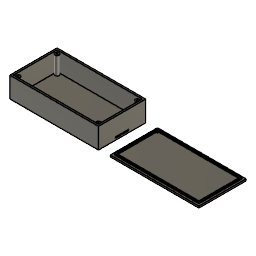
caja sensor examen (Autodesk Fusion 360 design; units mm, degrees)
part number: 2026-07-09-18-08-44-658
Autodesk Fusion 360 part; units mm, degrees
note: some values were not read from the file. Chosen so that the rebuilt part matches the saved one: which bodies a step acts on.
sketch "Boceto1" plane through (0, 0, 0) normal (0, 0, 1) x (1, 0, 0)
  line L0 (0, 0) -> (150, 0)
  line L1 (150, 0) -> (150, 80)
  line L2 (150, 80) -> (0, 80)
  line L3 (0, 80) -> (0, 0)
extrude "Extruir1" add sketch "Boceto1" along normal blind 3 makes body 1
sketch "Boceto2" plane through (0, 0, 0) normal (0, 0, 1) x (1, 0, 0)
  line L0 (0, 0) -> (150, 0)
  line L1 (150, 0) -> (150, 3)
  line L2 (150, 3) -> (0, 3)
  line L3 (0, 3) -> (0, 0)
extrude "Extruir2" add sketch "Boceto2" along normal blind 32 separate body makes body 2
move_body "Desplazar1" bodies 2 to x (1, 0, 0) y (0, 1, 0) z (0, 0, 1) at (0, 0, 3)
sketch "Boceto3" plane through (0, 0, 0) normal (0, 0, 1) x (1, 0, 0)
  line L0 (0, 77) -> (150, 77)
  line L1 (150, 77) -> (150, 80)
  line L2 (150, 80) -> (0, 80)
  line L3 (0, 80) -> (0, 77)
extrude "Extruir3" add sketch "Boceto3" along normal blind 32 separate body makes body 3
move_body "Desplazar2" bodies 3 to x (1, 0, 0) y (0, 1, 0) z (0, 0, 1) at (0, 0, 3)
sketch "Boceto4" plane through (0, 0, 0) normal (0, 0, 1) x (1, 0, 0)
  line L0 (0, 0) -> (3, 0)
  line L1 (3, 0) -> (3, 80)
  line L2 (3, 80) -> (0, 80)
  line L3 (0, 80) -> (0, 0)
extrude "Extruir4" add sketch "Boceto4" along normal blind 32 separate body makes body 4
move_body "Desplazar3" bodies 4 to x (1, 0, 0) y (0, 1, 0) z (0, 0, 1) at (0, 0, 3)
sketch "Boceto5" plane through (0, 0, 0) normal (0, 0, 1) x (1, 0, 0)
  line L0 (147, 0) -> (150, 0)
  line L1 (150, 0) -> (150, 29)
  line L2 (150, 29) -> (147, 29)
  line L3 (147, 29) -> (147, 0)
extrude "Extruir5" add sketch "Boceto5" along normal blind 32 separate body makes body 5
move_body "Desplazar4" bodies 5 to x (1, 0, 0) y (0, 1, 0) z (0, 0, 1) at (0, 0, 3)
sketch "Boceto6" plane through (0, 0, 0) normal (0, 0, 1) x (1, 0, 0)
  line L0 (147, 39) -> (150, 39)
  line L1 (150, 39) -> (150, 41)
  line L2 (150, 41) -> (147, 41)
  line L3 (147, 41) -> (147, 39)
extrude "Extruir6" add sketch "Boceto6" along normal blind 2 separate body makes body 6
move_body "Desplazar5" bodies 6 to x (1, 0, 0) y (0, 1, 0) z (0, 0, 1) at (0, 0, 3)
sketch "Boceto7" plane through (0, 0, 0) normal (0, 0, 1) x (1, 0, 0)
  line L0 (147, 51) -> (150, 51)
  line L1 (150, 51) -> (150, 80)
  line L2 (150, 80) -> (147, 80)
  line L3 (147, 80) -> (147, 51)
extrude "Extruir7" add sketch "Boceto7" along normal blind 32 separate body makes body 7
move_body "Desplazar6" bodies 7 to x (1, 0, 0) y (0, 1, 0) z (0, 0, 1) at (0, 0, 3)
sketch "Boceto8" plane through (0, 0, 0) normal (0, 0, 1) x (1, 0, 0)
  line L0 (147, 29) -> (150, 29)
  line L1 (150, 29) -> (150, 51)
  line L2 (150, 51) -> (147, 51)
  line L3 (147, 51) -> (147, 29)
extrude "Extruir8" add sketch "Boceto8" along normal blind 30 separate body makes body 8
move_body "Desplazar7" bodies 8 to x (1, 0, 0) y (0, 1, 0) z (0, 0, 1) at (0, 0, 5)
sketch "Boceto9" plane through (0, 0, 0) normal (0, 0, 1) x (1, 0, 0)
  circle A0 centre (7, 7) radius 3.5
extrude "Extruir9" add sketch "Boceto9" along normal blind 30 separate body makes body 9
move_body "Desplazar8" bodies 9 to x (1, 0, 0) y (0, 1, 0) z (0, 0, 1) at (0, 0, 3)
sketch "Boceto10" plane through (0, 0, 0) normal (0, 0, 1) x (1, 0, 0)
  circle A0 centre (7, 7) radius 1.1
extrude "Extruir10" cut sketch "Boceto10" along normal blind 37 bodies 1 9
sketch "Boceto11" plane through (0, 0, 0) normal (0, 0, 1) x (1, 0, 0)
  circle A0 centre (143, 7) radius 3.5
extrude "Extruir11" add sketch "Boceto11" along normal blind 30 separate body makes body 10
move_body "Desplazar9" bodies 10 to x (1, 0, 0) y (0, 1, 0) z (0, 0, 1) at (0, 0, 3)
sketch "Boceto12" plane through (0, 0, 0) normal (0, 0, 1) x (1, 0, 0)
  circle A0 centre (143, 7) radius 1.1
extrude "Extruir12" cut sketch "Boceto12" along normal blind 37 bodies 1 10
sketch "Boceto13" plane through (0, 0, 0) normal (0, 0, 1) x (1, 0, 0)
  circle A0 centre (7, 73) radius 3.5
extrude "Extruir13" add sketch "Boceto13" along normal blind 30 separate body makes body 11
move_body "Desplazar10" bodies 11 to x (1, 0, 0) y (0, 1, 0) z (0, 0, 1) at (0, 0, 3)
sketch "Boceto14" plane through (0, 0, 0) normal (0, 0, 1) x (1, 0, 0)
  circle A0 centre (7, 73) radius 1.1
extrude "Extruir14" cut sketch "Boceto14" along normal blind 37 bodies 1 11
sketch "Boceto15" plane through (0, 0, 0) normal (0, 0, 1) x (1, 0, 0)
  circle A0 centre (143, 73) radius 3.5
extrude "Extruir15" add sketch "Boceto15" along normal blind 30 separate body makes body 12
move_body "Desplazar11" bodies 12 to x (1, 0, 0) y (0, 1, 0) z (0, 0, 1) at (0, 0, 3)
sketch "Boceto16" plane through (0, 0, 0) normal (0, 0, 1) x (1, 0, 0)
  circle A0 centre (143, 73) radius 1.1
extrude "Extruir16" cut sketch "Boceto16" along normal blind 37 bodies 1 12
sketch "Boceto17" plane through (0, 0, 0) normal (0, 0, 1) x (1, 0, 0)
  line L0 (170, 0) -> (320, 0)
  line L1 (320, 0) -> (320, 80)
  line L2 (320, 80) -> (170, 80)
  line L3 (170, 80) -> (170, 0)
extrude "Extruir17" add sketch "Boceto17" along normal blind 3 separate body makes body 13
sketch "Boceto18" plane through (0, 0, 0) normal (0, 0, 1) x (1, 0, 0)
  line L0 (173.5, 3.5) -> (316.5, 3.5)
  line L1 (316.5, 3.5) -> (316.5, 5.5)
  line L2 (316.5, 5.5) -> (173.5, 5.5)
  line L3 (173.5, 5.5) -> (173.5, 3.5)
extrude "Extruir18" add sketch "Boceto18" along normal blind 2 separate body makes body 14
move_body "Desplazar12" bodies 14 to x (1, 0, 0) y (0, 1, 0) z (0, 0, 1) at (0, 0, 3)
sketch "Boceto19" plane through (0, 0, 0) normal (0, 0, 1) x (1, 0, 0)
  line L0 (173.5, 74.5) -> (316.5, 74.5)
  line L1 (316.5, 74.5) -> (316.5, 76.5)
  line L2 (316.5, 76.5) -> (173.5, 76.5)
  line L3 (173.5, 76.5) -> (173.5, 74.5)
extrude "Extruir19" add sketch "Boceto19" along normal blind 2 separate body makes body 15
move_body "Desplazar13" bodies 15 to x (1, 0, 0) y (0, 1, 0) z (0, 0, 1) at (0, 0, 3)
sketch "Boceto20" plane through (0, 0, 0) normal (0, 0, 1) x (1, 0, 0)
  line L0 (173.5, 3.5) -> (175.5, 3.5)
  line L1 (175.5, 3.5) -> (175.5, 76.5)
  line L2 (175.5, 76.5) -> (173.5, 76.5)
  line L3 (173.5, 76.5) -> (173.5, 3.5)
extrude "Extruir20" add sketch "Boceto20" along normal blind 2 separate body makes body 16
move_body "Desplazar14" bodies 16 to x (1, 0, 0) y (0, 1, 0) z (0, 0, 1) at (0, 0, 3)
sketch "Boceto21" plane through (0, 0, 0) normal (0, 0, 1) x (1, 0, 0)
  line L0 (314.5, 3.5) -> (316.5, 3.5)
  line L1 (316.5, 3.5) -> (316.5, 76.5)
  line L2 (316.5, 76.5) -> (314.5, 76.5)
  line L3 (314.5, 76.5) -> (314.5, 3.5)
extrude "Extruir21" add sketch "Boceto21" along normal blind 2 separate body makes body 17
move_body "Desplazar15" bodies 17 to x (1, 0, 0) y (0, 1, 0) z (0, 0, 1) at (0, 0, 3)
sketch "Boceto22" plane through (0, 0, 0) normal (0, 0, 1) x (1, 0, 0)
  circle A0 centre (177, 7) radius 1.1
extrude "Extruir22" cut sketch "Boceto22" along normal blind 5 bodies 13
sketch "Boceto23" plane through (0, 0, 0) normal (0, 0, 1) x (1, 0, 0)
  circle A0 centre (313, 7) radius 1.1
extrude "Extruir23" cut sketch "Boceto23" along normal blind 5 bodies 13
sketch "Boceto24" plane through (0, 0, 0) normal (0, 0, 1) x (1, 0, 0)
  circle A0 centre (177, 73) radius 1.1
extrude "Extruir24" cut sketch "Boceto24" along normal blind 5 bodies 13
sketch "Boceto25" plane through (0, 0, 0) normal (0, 0, 1) x (1, 0, 0)
  circle A0 centre (313, 73) radius 1.1
extrude "Extruir25" cut sketch "Boceto25" along normal blind 5 bodies 13
combine "Combinar1" operation add target body 3 tool bodies 4 2 5 6 7 9 10 8 12 11 makes body 18 at (140.5562, 9.5055, 23) makes body 19 at (145.3159, 75.6242, 23) makes body 20 at (10.4826, 6.6515, 23) makes body 21 at (10.2252, 71.6405, 23)
combine "Combinar2" operation add target body 1 tool bodies 3 18 19 20 21
combine "Combinar3" operation add target body 17 tool bodies 16 15 14 13
named bodies: "Piso liso caja", "Pared lateral 1", "Pared lateral 2", "Pared frontal cerrada", "Pared sensor izquierda", "Separador sensor central", "Pared sensor derecha", "Puente superior sensor", "Poste tornillo tapa", "Poste tornillo tapa (1)", "Poste tornillo tapa (2)", "Poste tornillo tapa (3)", "Tapa superior lisa sin LED", "Labio tapa inferior", "Labio tapa superior", "Labio tapa izquierdo", "Labio tapa derecho", "Pared lateral 2 (1)", "Pared lateral 2 (2)", "Pared lateral 2 (3)", "Pared lateral 2 (4)"
